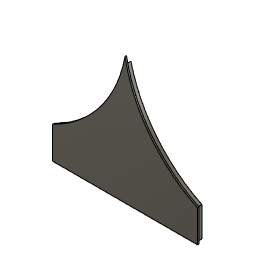
Ramp for Checkers v1 (Autodesk Fusion 360 design; units mm, degrees)
Autodesk Fusion 360 part; units mm, degrees
sketch "Sketch1" plane through (0, 0, 0) normal (0, 0, 1) x (1, 0, 0)
  line L0 (0, 0) -> (0, 254) construction
  line L1 (0, 0) -> (152.4, 0)
  line L2 (152.4, 0) -> (152.4, 63.5)
  arc A0 (0, 254) -> (152.4, 63.5) centre (278.7714, 320.8071) ccw
  arc A1 (-152.4, 63.5) -> (0, 254) centre (-278.7714, 320.8071) ccw
  line L3 (-152.4, 0) -> (-152.4, 63.5)
  line L4 (0, 0) -> (-152.4, 0)
  dimension "d1" = 254
  dimension "d2" = 152.4
  dimension "d3" = 63.5
  constraint coincident L0.start L1.start
  constraint vertical L0
  constraint perpendicular L0 L1
  constraint perpendicular L1 L2
  constraint symmetric A0.start L0 A1.end
  constraint symmetric L0 L1.start L4.start
  constraint symmetric L0 L1.end L3.start
  constraint symmetric L0 L2.end A1.start
  constraint symmetric L0 A0 A1
  measures "d1" distance of L0.start L0.end
  measures "d2" distance of L0.start L1.end
  measures "d3" distance of L1.end L2.end
extrude "Extrude1" add sketch "Sketch1" along normal blind 9.525
sketch "Sketch2" plane through (0, 0, 9.525) normal (0, 0, 1) x (1, 0, 0)
  line L0 (152.4, 0) -> (152.4, 63.5)
  arc A0 (0, 254) -> (152.4, 63.5) centre (278.7714, 320.8071) ccw
  arc A1 (-152.4, 63.5) -> (0, 254) centre (-278.7714, 320.8071) ccw
  line L1 (-152.4, 63.5) -> (-152.4, 0)
  line L2 (-152.4, 0) -> (152.4, 0)
  line L3 (155.575, -3.175) -> (155.575, 65.4856)
  arc A2 (0, 269.3003) -> (155.575, 65.4856) centre (278.7714, 320.8071) ccw
  arc A3 (-155.575, 65.4856) -> (0, 269.3003) centre (-278.7714, 320.8071) ccw
  line L4 (-155.575, 65.4856) -> (-155.575, -3.175)
  line L5 (-155.575, -3.175) -> (155.575, -3.175)
  dimension "d6" = -3.175
extrude "Extrude2" add sketch "Sketch2" along normal blind 3.175 contours L0 A0 A1 L1 L2 | L3 A2 A3 L4 L5
equation "d1 = 10\""
equation "d2 = 6\""
